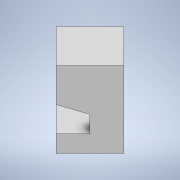
# Autodesk Inventor part: Деталь1Индивидуал
Saved by Autodesk Inventor 2021.1 (Build 251245010, 245A)
## iProperties
Created: 2023-10-12
Part Number: Деталь1Индивидуал
Material: Типовые
Document SubType Name: Modeling
Designer: Lenovo
Density: 1 g/cm^3
Appearance: По умолчанию
Author: Lenovo
Autodesk Inventor part; units mm, degrees
ref_plane "YZ Plane" through (0, 0, 0) normal (1, 0, 0) x (0, 1, 0)
ref_plane "XZ Plane" through (0, 0, 0) normal (0, 1, 0) x (-1, 0, 0)
ref_plane "XY Plane" through (0, 0, 0) normal (0, 0, 1) x (1, 0, 0)
sketch "Эскиз1" plane through (0, 0, 0) normal (0, 1, 0) x (-1, 0, 0)
  circle A0 centre (0, 0) radius 40
  line L0 (0, 40) -> (40, 0)
  line L1 (40, 0) -> (0, -40)
  line L2 (0, -40) -> (-40, 0)
  line L3 (-40, 0) -> (0, 40)
  dimension "d0" = 80
  constraints: 8 end point, 2 coincident, 1 vertical alignment, 11 other
extrude "Выдавливание1" add sketch "Эскиз1" along normal blind 90 contours L1 L2 L3 L0
sketch "Эскиз2" plane through (0, 0, 0) normal (0, 0, 1) x (1, 0, 0)
  line L0 (0, 90) -> (-40, 90) projected
  line L1 (-40, 90) -> (-40, 70)
  line L2 (-40, 0) -> (-40, 90) projected
  line L3 (0, 0) -> (-40, 0) projected
  line L4 (-40, 0) -> (-40, 20)
  line L5 (-40, 20) -> (20, 20)
  line L6 (20, 20) -> (20, 40)
  line L7 (20, 40) -> (-40, 70)
  line L8 (-40, 20) -> (-40, 70)
  dimension "d3" = 20
  dimension "d4" = 20
  dimension "d5" = 60
  dimension "d6" = 20
  constraints: 12 end point, 2 perpendicular, 2 point on line, 1 parallel
  measures "d3" distance of L0.end L1.end
  measures "d4" distance of L2.start L4.end
  measures "d5" distance of L4.end L5.end
  measures "d6" distance of L5.end L6.end
extrude "Выдавливание2" cut sketch "Эскиз2" against normal mid plane 90
